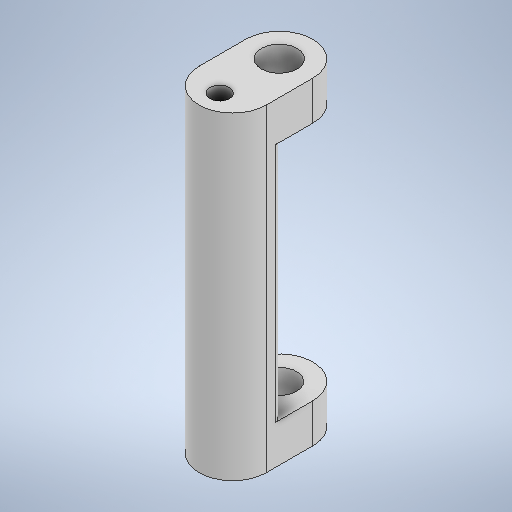
# Autodesk Inventor part: Odometer_Test_Bracket
Saved by Autodesk Inventor 2025.1 (Build 291241020, 241B)
## iProperties
Created: 2024-11-14
Part Number: Odometer_Test_Bracket
Material: Generic
Document SubType Name: Modeling
Designer: AtuStem
Density: 1 g/cm^3
Appearance: Default
Author: AtuStem
Autodesk Inventor part; units mm, degrees
ref_plane "YZ Plane" through (0, 0, 0) normal (1, 0, 0) x (0, 1, 0)
ref_plane "XZ Plane" through (0, 0, 0) normal (0, 1, 0) x (-1, 0, 0)
ref_plane "Work Plane7" through (0, 5.08, 0) normal (0, 1, 0) x (1, 0, 0)
sketch "Sketch3" plane through (0, 5.08, 0) normal (0, 1, 0) x (1, 0, 0)
  circle A0 centre (0, 0) radius 6.5659 projected
  circle A1 centre (0, 0) radius 3.3655 projected
  line L0 (-6.5659, 0) -> (-6.5659, -6.5683)
  line L1 (-6.5659, -6.5683) -> (6.5659, -6.5683)
  line L2 (6.5659, -6.5683) -> (6.5659, 0)
  line L3 (0, -6.5683) -> (0, -9.1083)
  line L4 (0, 0) -> (0, -9.1083) construction
  line L5 (6.5659, 0) -> (6.5659, -9.1083)
  line L6 (-6.5659, -9.1083) -> (-6.5659, 0)
  arc A2 (6.5659, 0) -> (-6.5659, 0) centre (0, 0) ccw
  arc A3 (-6.5659, -9.1083) -> (6.5659, -9.1083) centre (0, -9.1083) ccw
  line L7 (0, -6.5683) -> (0, -7.8383)
  arc A4 (-6.5659, -4.2811) -> (6.5659, -4.2811) centre (0, 0) ccw
  point P0 (0, -4.5541)
  dimension "d19" = 2.54
  dimension "d20" = 1.27
  constraints: 18 end point, 9 point on circle, 5 tangent, 3 centre point, 3 point on line, 3 vertical, 2 midpoint, 1 coincident, 1 parallel, 1 perpendicular
  measures "d19" distance of L3.start L3.end
  measures "d20" distance of L3.start L7.end
extrude "Extrusion5" add sketch "Sketch3" along normal blind 2.54 contours A0 | L2 A4 L1 L0 A0 | L2 L1 A4 | A4 L1 L0 | L5 A3 L6 L1 A4 | A4 L3 L1 | L1 L3 A4 | A1
extrude "Extrusion6" add sketch "Sketch3" along normal blind 7.62
sketch "Sketch4" plane through (0, 12.7, 0) normal (0, 1, 0) x (1, 0, 0)
  line L0 (-6.5659, 0) -> (-6.5659, -9.1083) projected
  arc A0 (-6.5659, -9.1083) -> (6.5659, -9.1083) centre (0, -9.1083) ccw projected
  line L1 (6.5659, -9.1083) -> (6.5659, 0) projected
  arc A1 (6.5659, 0) -> (-6.5659, 0) centre (0, 0) ccw projected
  circle A2 centre (0, 0) radius 3.3655 projected
  line L2 (0, -3.3655) -> (0, -7.1755)
  line L3 (0, -7.1755) -> (6.5659, -7.1755)
  line L4 (0, -7.1755) -> (-6.5659, -7.1755)
  arc A3 (-6.5659, -2.8943) -> (6.5659, -2.8943) centre (0, 0) ccw
  line L5 (0, -9.1083) -> (0, -7.1755)
  line L6 (0, -7.1755) -> (0, -7.8105)
  arc A4 (-6.5659, -4.23) -> (6.5659, -4.23) centre (0, 0) ccw
  dimension "d25" = 3.81
  dimension "d27" = 0.635
  constraints: 10 end point, 8 point on line, 6 point on circle, 2 centre point, 2 coincident, 2 perpendicular, 1 vertical, 1 vertical alignment, 1 other
  measures "d25" distance of L2.start L2.end
  measures "d27" distance of L2.end L6.end
extrude "Extrusion7" add sketch "Sketch4" along normal blind 52.07 contours A4 L4 L0 | L4 A4 L3 L1 A0 L0 | A4 L1 L3
fillet "Fillet1" radius 1.27 2 edges at (6.5659, 38.735, 4.23) (-6.5659, 38.735, 4.23)
sketch "Sketch5" plane through (0, 64.77, 0) normal (0, 1, 0) x (1, 0, 0)
  arc A0 (-4.5552, -6.3446) -> (-6.5659, -7.3762) centre (-5.2959, -7.3762) ccw projected
  line L0 (-6.5659, -7.3762) -> (-6.5659, -9.1083) projected
  arc A1 (-6.5659, -9.1083) -> (6.5659, -9.1083) centre (0, -9.1083) ccw projected
  line L1 (6.5659, -9.1083) -> (6.5659, -7.3762) projected
  arc A2 (6.5659, -7.3762) -> (4.5552, -6.3446) centre (5.2959, -7.3762) ccw projected
  arc A3 (-4.5552, -6.3446) -> (4.5552, -6.3446) centre (0, 0) ccw projected
  arc A4 (-4.5552, -6.3446) -> (4.5552, -6.3446) centre (0, 0) ccw projected
  arc A5 (6.5659, -7.3762) -> (4.5552, -6.3446) centre (5.2959, -7.3762) ccw projected
  line L2 (6.5659, -7.3762) -> (6.5659, 0) projected
  arc A6 (6.5659, 0) -> (-6.5659, 0) centre (0, 0) ccw projected
  line L3 (-6.5659, 0) -> (-6.5659, -7.3762) projected
  arc A7 (-4.5552, -6.3446) -> (-6.5659, -7.3762) centre (-5.2959, -7.3762) ccw projected
  circle A8 centre (0, 0) radius 3.3655 projected
  circle A9 centre (0, 0) radius 3.4925
  line L4 (0, -9.1083) -> (0, -11.0133)
  line L5 (5.2959, -7.3762) -> (0, -11.0133)
  line L6 (-5.2959, -7.3762) -> (0, -11.0133)
  line L7 (0, -11.0133) -> (0, -11.6483)
  circle A10 centre (0, -11.6483) radius 1.905
  point P0 (6.5659, -7.3762)
  dimension "d31" = 6.985
  dimension "d32" = 1.905
  dimension "d34" = 0.635
  dimension "d35" = 3.81
  constraints: 8 end point, 2 centre point, 2 coincident, 2 vertical
  measures "d31" diameter of A9
  measures "d32" distance of L4.start L4.end
  measures "d34" distance of L4.end L7.end
  measures "d35" diameter of A10
extrude "Extrusion8" add sketch "Sketch5" along normal blind 7.62 contours A3 A2 L1 A1 L0 A0 | A0 L3 A6 L2 A2 A3
extrude "Extrusion9" cut sketch "Sketch5" against normal blind 7.62 contours A10 L5 L4 | L4 L6 A10 | L5 A10 L6
sketch "Sketch6" plane through (0, 72.39, 0) normal (0, 1, 0) x (1, 0, 0)
  arc A0 (6.5659, 0) -> (-6.5659, 0) centre (0, 0) ccw projected
  line L0 (-6.5659, 0) -> (-6.5659, -9.1083) projected
  arc A1 (-6.5659, -9.1083) -> (6.5659, -9.1083) centre (0, -9.1083) ccw projected
  line L1 (6.5659, -9.1083) -> (6.5659, 0) projected
  circle A2 centre (0, -11.6483) radius 1.905 projected
  circle A3 centre (0, 0) radius 3.4925 projected
extrude "Extrusion10" add sketch "Sketch6" against normal blind 12.7
extrude "Extrusion11" cut sketch "Sketch6" against normal blind 5.08
sketch "Sketch7" plane through (0, 57.15, 11.6483) normal (0, 1, 0) x (1, 0, 0)
  circle A0 centre (0, 0) radius 1.905 projected
  point P0 (0, 11.6483)
extrude "Extrusion12" add sketch "Sketch7" along normal blind 2.54
body "Solid3"
